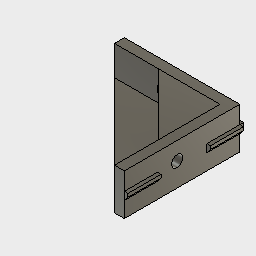
CornerBrace (Autodesk Fusion 360 design; units mm, degrees)
Autodesk Fusion 360 part; units mm, degrees
sketch "Sketch1" plane through (0, 0, 0) normal (0, 0, 1) x (1, 0, 0) in component "CornerBrace (1)"
  line L0 (82.6456, 31.4944) -> (82.6456, -3.4575)
  line L1 (82.6456, -3.4575) -> (79.6456, -3.4575)
  line L2 (79.6456, -3.4575) -> (70.444, 5.744)
  line L3 (70.444, 5.744) -> (47.6981, 28.4944)
  line L4 (47.6981, 28.4944) -> (47.6981, 31.4944)
  line L5 (47.6981, 31.4944) -> (82.6456, 31.4944)
  line L6 (79.6456, -3.4575) -> (79.6456, 28.4944)
  line L7 (79.6456, 28.4944) -> (47.6981, 28.4944)
  dimension "d163_1" = 3
  dimension "d164_1" = 3
  constraint vertical L0
  constraint perpendicular L0 L1
  constraint vertical L4
  constraint perpendicular L1 L6
  constraint horizontal L5
  constraint parallel L5 L7
  measures "d163_1" distance of L5 L7
  measures "d164_1" distance of L0 L6
extrude "Extrude1" add sketch "Sketch1" along normal blind 12.5 contours L0 L1 L4 L5 L6 L7 makes body 1 in component "CornerBrace (1)"
extrude "Extrude2" add sketch "Sketch1" along normal blind 3.5 contours L2 L3 L6 L7 bodies 1 in component "CornerBrace (1)"
sketch "Sketch2" plane through (0, 28.4944, 0) normal (0, -1, 0) x (1, 0, 0) in component "CornerBrace (1)"
  line L0 (47.6981, 3.5) -> (79.6456, 3.5) construction
  line L1 (79.6456, 3.5) -> (79.6456, 12.5)
  line L2 (79.6456, 12.5) -> (47.6981, 12.5) construction
  line L3 (47.6981, 12.5) -> (47.6981, 3.5)
  circle A0 centre (63.6981, 7.09) radius 1.7
  circle A1 centre (63.6981, 7.09) radius 3
  dimension "d175_1" = 3.4
  dimension "d178_1" = 1.3
  dimension "d179_1" = 16
  dimension "d207" = 3.59
  constraint midpoint L3
  constraint midpoint L0
  measures "d175_1" diameter of A0
sketch "Sketch3" plane through (79.6456, 0, 0) normal (-1, 0, 0) x (0, -1, 0) in component "CornerBrace (1)"
  line L0 (-28.4944, 3.5) -> (3.4575, 3.5)
  line L1 (3.4575, 3.5) -> (3.4575, 12.5)
  line L2 (3.4575, 12.5) -> (-28.4944, 12.5)
  line L3 (-28.4944, 12.5) -> (-28.4944, 3.5)
  circle A0 centre (-12.5425, 7.09) radius 1.7
  circle A1 centre (-12.5425, 7.09) radius 3
  dimension "d176_1" = 3.4
  dimension "d177_1" = 1.3
  dimension "d181_1" = 16
  dimension "d208" = 3.59
  constraint midpoint L1
  measures "d176_1" diameter of A0
  measures "d208" distance of L0
extrude "Extrude3" cut sketch "Sketch2" against normal blind 0.5 bodies 1 in component "CornerBrace (1)"
extrude "Extrude4" cut sketch "Sketch2" against normal up to surface (3 mm away) contours A0 bodies 1 in component "CornerBrace (1)"
extrude "Extrude5" cut sketch "Sketch3" against normal blind 0.5 contours A1 bodies 1 in component "CornerBrace (1)"
extrude "Extrude6" cut sketch "Sketch3" against normal up to surface (3 mm away) contours A0 bodies 1 in component "CornerBrace (1)"
sketch "Sketch5" plane through (0, -3.4575, 0) normal (0, -1, 0) x (1, 0, 0) in component "CornerBrace (1)"
  line L0 (79.6456, 0) -> (82.6456, 0)
  line L1 (82.6456, 0) -> (82.6456, 12.5)
  line L2 (82.6456, 12.5) -> (79.6456, 12.5)
  line L3 (79.6456, 12.5) -> (79.6456, 3.5)
  line L4 (79.6456, 3.5) -> (79.6456, 0)
  line L5 (82.6456, 7.1528) -> (82.6456, 4.7528)
  line L6 (82.6456, 7.1528) -> (83.7456, 7.1528)
  line L7 (83.7456, 7.1528) -> (83.7456, 6.1528)
  line L8 (83.7456, 6.1528) -> (82.6456, 4.7528)
  dimension "d189_1" = 2.4
  dimension "d190_1" = 1.1
  dimension "d191_1" = 1
  constraint coincident L1
  constraint parallel L1 L5
  constraint perpendicular L5 L6
extrude "Extrude7" add sketch "Sketch5" against normal blind 10 separate body contours L1 L5 L6 L7 L8 makes body 2 in component "CornerBrace (1)"
copy_body "CopyPasteBodies1" bodies 2 makes body 3 in component "CornerBrace (1)"
move_body "MoveBody1" bodies 3 to x (1, 0, 0) y (0, 1, 0) z (0, 0, 1) at (0, 25, 0) in component "CornerBrace (1)"
copy_body "CopyPasteBodies2" bodies 2 makes body 4 in component "CornerBrace (1)"
move_body "MoveBody2" bodies 4 to x (0, 1, 0) y (-1, 0, 0) z (0, 0, 1) at (79.1881, -51.1032, 0) in component "CornerBrace (1)"
copy_body "CopyPasteBodies3" bodies 4 makes body 5 in component "CornerBrace (1)"
move_body "MoveBody3" bodies 5 to x (1, 0, 0) y (0, 1, 0) z (0, 0, 1) at (-25, 0, 0) in component "CornerBrace (1)"
sketch "Sketch6" plane through (0, 0, 12.5) normal (0, 0, 1) x (-1, 0, 0) in component "CornerBrace (1)"
  line L0 (-79.6456, -28.4944) -> (-79.6456, 3.4575)
  line L1 (-79.6456, 3.4575) -> (-82.6456, 3.4575)
  line L2 (-82.6456, 3.4575) -> (-82.6456, -31.4944)
  line L3 (-82.6456, -31.4944) -> (-47.6981, -31.4944)
  line L4 (-47.6981, -31.4944) -> (-47.6981, -28.4944)
  line L5 (-47.6981, -28.4944) -> (-79.6456, -28.4944)
  line L6 (-79.6456, -31.4944) -> (-79.6456, -9.9944)
  line L7 (-79.6456, -31.4944) -> (-101.1456, -31.4944) construction
  line L8 (-82.6456, -28.4944) -> (-61.1456, -28.4944)
  line L9 (-61.1456, -28.4944) -> (-79.6456, -9.9944)
  dimension "d194" = 90
  dimension "d195" = 21.5
  dimension "d196" = 21.5
  constraint coincident L3
  constraint horizontal L7
  constraint coincident L2
  constraint coincident L5
  constraint perpendicular L2 L8
  measures "d194" angle of L6 L7
extrude "Extrude8" add sketch "Sketch6" against normal blind 7 separate body contours L0 L5 L6 L8 L9 makes body 6 in component "CornerBrace (1)"
sketch "Sketch9" plane through (44.82, 44.82, 0) normal (-0.707107, -0.707107, 0) x (0.707107, -0.707107, 0) in component "CornerBrace (1)"
  line L0 (49.2509, 12.5) -> (23.0879, 12.5)
  line L1 (23.0879, 12.5) -> (23.0879, 5.5)
  line L2 (23.0879, 5.5) -> (49.2509, 5.5)
  line L3 (49.2509, 5.5) -> (49.2509, 12.5)
  line L4 (23.0879, 12.5) -> (23.0879, 10.5)
  line L5 (49.2509, 12.5) -> (49.2509, 5.5)
  line L6 (23.0879, 10.5) -> (49.2509, 10.506)
  dimension "d201" = 2
  constraint parallel L1 L4
  constraint coincident L3
ref_plane "WorkPlane1" through (70.3956, 19.2444, 10.503) normal (0.206582, 0.206894, 0.956305) x (0.707107, -0.707107, 0.00023) in component "CornerBrace (1)"
sketch "Sketch10" plane through (70.5932, 19.4422, 10.4175) normal (0.206582, 0.206894, 0.956305) x (0.707107, -0.707107, 0.00023) in component "CornerBrace (1)"
sketch "Sketch12" plane through (70.5932, 19.4422, 10.4175) normal (0.206582, 0.206894, 0.956305) x (0.707107, -0.707107, 0.00023) in component "CornerBrace (1)"
  line L0 (13.0817, -0.2924) -> (-0.0009, 13.6802)
  line L1 (-0.0009, 13.6802) -> (-13.0812, -0.2924)
  line L2 (-13.0812, -0.2924) -> (13.0817, -0.2924)
  line L3 (40.7563, -12.2924) -> (-0.0017, 31.2384)
  line L4 (-0.0017, 31.2384) -> (-40.7526, -12.2924)
  line L5 (-40.7526, -12.2924) -> (40.7563, -12.2924)
  dimension "d203" = 12
  measures "d203" distance of L0
extrude "Extrude9" cut sketch "Sketch12" against normal blind 6 contours L0 L1 L2 | L3 L4 L5 bodies 6 in component "CornerBrace (1)"
component "CornerBrace (1)" placed x (1, 0, 0) y (0, 1, 0) z (0, 0, 1) at (125, 0, 0)
equation "d196 = d195"
